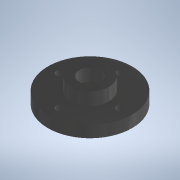
# Autodesk Inventor part: SERVOHORN
Saved by Autodesk Inventor 2021 (Build 250183000, 183)
## iProperties
Created: 2017-08-15
Part Number: SERVOHORN
Material: Generic
Document SubType Name: Modeling
Designer: Izuwa
Density: 1 g/cm^3
Appearance: Default
Mass: 0.939164 g
Surface Area: 9.86284 cm^2
Volume: 0.939164 cm^3
Author: Izuwa
Autodesk Inventor part; units mm, degrees
ref_plane "YZ Plane" through (0, 0, 0) normal (1, 0, 0) x (0, 1, 0)
ref_plane "XZ Plane" through (0, 0, 0) normal (0, 1, 0) x (-1, 0, 0)
ref_plane "XY Plane" through (0, 0, 0) normal (0, 0, 1) x (1, 0, 0)
sketch "Sketch1" plane through (0, 0, 0) normal (0, 0, 1) x (1, 0, 0)
  circle A0 centre (0, 0) radius 10
  dimension "d0" = 20
  constraints: 1 centre point, 1 coincident
  measures "d0" diameter of A0
extrude "Extrusion1" add sketch "Sketch1" along normal blind 2.77
sketch "Sketch2" plane through (0, 0, 2.77) normal (0, 0, 1) x (1, 0, 0)
  circle A0 centre (0, 0) radius 2.5
  circle A1 centre (0, 0) radius 4.5
  dimension "d3" = 5
  dimension "d4" = 9
  constraints: 2 centre point, 2 coincident
  measures "d3" diameter of A0
  measures "d4" diameter of A1
extrude "Extrusion2" add sketch "Sketch2" along normal blind 3
sketch "Sketch3" plane through (0, 0, 0) normal (0, 0, -1) x (-1, 0, 0)
  circle A0 centre (7.2, 0) radius 0.9
  circle A1 centre (0, 7.2) radius 0.9
  circle A2 centre (-7.2, 0) radius 0.9
  circle A3 centre (0, -7.2) radius 0.9
  point P0 (0, 0)
  dimension "d11" = 360
  constraints: 4 centre point, 9 other
extrude "Extrusion3" cut sketch "Sketch3" against normal blind 3
sketch "Sketch4" plane through (0, 0, 0) normal (0, 0, -1) x (-1, 0, 0)
  circle A0 centre (0, 0) radius 2
  dimension "d18" = 4
  constraints: 1 centre point, 1 coincident
  measures "d18" diameter of A0
extrude "Extrusion4" cut sketch "Sketch4" against normal blind 5
sketch "Sketch5" plane through (0, 0, 0) normal (0, 0, -1) x (-1, 0, 0)
  point P0 (0, 0)
equation "\"d16\" = d15"
equation "\"d15\" = 5"
body "Solid1"
